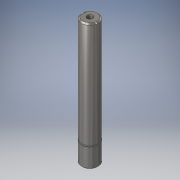
# Autodesk Inventor part: Drum_Axle
Saved by Autodesk Inventor 2016 (Build 200138000, 138)
## iProperties
Created: 2016-04-11
Part Number: Drum_Axle
Material: Steel, High Strength, Low Alloy
Document SubType Name: Modeling
Designer: agmle
Density: 7.85 g/cm^3
Appearance: Steel - Polished
Author: agmle
Autodesk Inventor part; units mm, degrees
ref_plane "YZ Plane" through (0, 0, 0) normal (1, 0, 0) x (0, 1, 0)
ref_plane "XZ Plane" through (0, 0, 0) normal (0, 1, 0) x (-1, 0, 0)
ref_plane "XY Plane" through (0, 0, 0) normal (0, 0, 1) x (1, 0, 0)
sketch "Sketch1" plane through (0, 0, 0) normal (0, 1, 0) x (-1, 0, 0)
  arc A0 (6.1484, 1.5875) -> (6.1484, -1.5875) centre (0, 0) ccw
  line L0 (6.1484, 1.5875) -> (4.5604, 1.5875)
  line L1 (4.5604, 1.5875) -> (4.5604, -1.5875)
  line L2 (4.5604, -1.5875) -> (6.1484, -1.5875)
  line L3 (4.5604, 0) -> (0, 0) construction
  dimension "d0" = 12.7
  dimension "d1" = 3.175
  dimension "d2" = 1.588
  constraints: 8 end point, 2 horizontal, 2 point on circle, 1 centre point, 1 coincident, 1 midpoint, 1 parallel, 1 perpendicular
  measures "d0" diameter of A0
  measures "d1" distance between parallel lines of L2 L0
  measures "d2" distance of L0.start L0.end
extrude "Extrusion1" add sketch "Sketch1" along normal blind 95.25
chamfer "Chamfer1" distance 1 angle 45 2 edges at (6.35, 0, 0) (6.35, 95.25, 0)
hole "Hole1" at (0, 0, 0) direction (0, 1, 0) diameter 4.2 depth 14 tip angle 118
hole "Hole2" at (0, 95.25, 0) direction (0, -1, 0) diameter 4.2 depth 14 tip angle 118
sketch "Sketch2" plane through (0, 0, 0) normal (0, 0, 1) x (1, 0, 0)
  line L0 (0, 0) -> (0, 95.25) construction
  line L1 (-2.1, 95.25) -> (2.1, 95.25) construction
  line L2 (-6.35, 14.775) -> (-6.0452, 14.775)
  line L3 (-6.0452, 14.775) -> (-6.0452, 15.875)
  line L4 (-6.0452, 15.875) -> (-6.35, 15.875)
  line L5 (-6.35, 15.875) -> (-6.35, 14.775)
  dimension "d30" = 1.1
  dimension "d32" = 6.35
  dimension "d33" = 79.375
  dimension "d38" = 6.0452
  constraints: 10 end point, 2 parallel, 1 horizontal, 1 midpoint, 1 perpendicular
  measures "d30" distance of L4.end L2.start
  measures "d32" distance between parallel lines of L0 L5
  measures "d33" distance from line of L1 L4.end
  measures "d38" distance between parallel lines of L0 L3
revolve "Revolution1" cut sketch "Sketch2" angle 360 about axis through (0, 0, 0) along (0, 1, 0)
body "Solid1"
